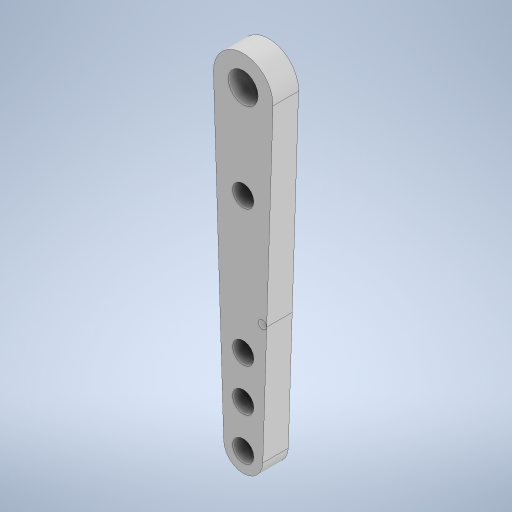
# Autodesk Inventor part: Hudson 1-65
Saved by Autodesk Inventor 2024.2 (Build 282272000, 272)
## iProperties
Created: 2024-10-09
Part Number: Hudson 1-65
Material: Genérico
Document SubType Name: Modeling
Designer: Monica Mora
Density: 1 g/cm^3
Appearance: Valor por defecto
Author: Monica Mora
Autodesk Inventor part; units mm, degrees
ref_plane "YZ Plane" through (0, 0, 0) normal (1, 0, 0) x (0, 1, 0)
ref_plane "XZ Plane" through (0, 0, 0) normal (0, 1, 0) x (-1, 0, 0)
ref_plane "XY Plane" through (0, 0, 0) normal (0, 0, 1) x (1, 0, 0)
sketch "Boceto1" plane through (0, 0, 0) normal (0, 0, 1) x (1, 0, 0)
  circle A0 centre (0, 0) radius 1.25
  arc A1 (-2.2988, -0.0746) -> (2.2988, -0.0746) centre (0, 0) ccw
  arc A2 (3.4982, 36.8865) -> (-3.4982, 36.8865) centre (0, 37) ccw
  circle A3 centre (0, 37) radius 1.75
  line L0 (0, 0) -> (0, 37) construction
  line L1 (-3.4982, 36.8865) -> (-2.2988, -0.0746)
  line L2 (3.4982, 36.8865) -> (2.2988, -0.0746)
  circle A4 centre (0, 5) radius 1.25
  circle A5 centre (0, 10) radius 1.25
  circle A6 centre (0, 26) radius 1.25
  circle A7 centre (2.2552, 14) radius 0.5
  point P0 (2.755, 13.9838)
  dimension "d0" = 37
  dimension "d1" = 7
  dimension "d2" = 3.5
  dimension "d3" = 4.6
  dimension "d4" = 2.5
  dimension "d5" = 2.5
  dimension "d6" = 2.5
  dimension "d7" = 2.5
  dimension "d8" = 5
  dimension "d9" = 5
  dimension "d10" = 4
  dimension "d11" = 1
  dimension "d12" = 12
  constraints: 8 centre point, 6 end point, 5 tangent, 4 coincident, 4 point on circle, 3 point on line, 1 vertical
  measures "d0" distance of L0.start L0.end
  measures "d1" diameter of A2
  measures "d2" diameter of A3
  measures "d3" diameter of A1
  measures "d4" diameter of A0
  measures "d5" diameter of A6
  measures "d6" diameter of A5
  measures "d7" diameter of A4
  measures "d8" distance of point (0, 0) A4.centre
  measures "d9" distance of A4.centre A5.centre
  measures "d10" vertical distance of A5.centre A7.centre
  measures "d11" diameter of A7
  measures "d12" vertical distance of A7.centre A6.centre
extrude "Extrusión1" add sketch "Boceto1" along normal blind 3
equation "\"d5\" = d4"
equation "\"d6\" = d4"
equation "\"d7\" = d4"
